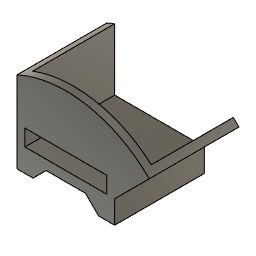
LED Mount Baffled Voron V0 V3D v7 (Autodesk Fusion 360 design; units mm, degrees)
Autodesk Fusion 360 part; units mm, degrees
note: some values were not read from the file. Set by a fixed rule: which sketch regions a step uses.
sketch "Sketch1" plane through (0, 0, 0) normal (0, 1, 0) x (1, 0, 0)
  line L0 (0, 0) -> (3, 0)
  line L1 (3, 0) -> (3, -16.2727) construction
  line L2 (9.25, -4) -> (-3.25, -4)
  line L3 (-3.25, -4) -> (-3.25, -1.5)
  line L4 (-3.25, -1.5) -> (9.25, -1.5)
  line L5 (9.25, -1.5) -> (9.25, -4)
  line L6 (9.25, -4) -> (-3.25, -1.5) construction
  line L7 (-3.25, -4) -> (9.25, -1.5) construction
  line L8 (0, 0) -> (-2, 2)
  line L9 (-2, 2) -> (-4.45, 2)
  line L10 (-4.45, 2) -> (-4.45, -1.5)
  line L11 (6, 0) -> (3, 0)
  line L12 (6, 0) -> (8, 2)
  line L13 (8, 2) -> (10.45, 2)
  line L14 (10.45, 2) -> (10.45, -1.5)
  line L15 (10.45, -1.5) -> (15.7279, -6.7779)
  arc A0 (-4.45, -10.4359) -> (15.7279, -6.7779) centre (3, 5.95) ccw
  line L16 (-4.45, -1.5) -> (-4.45, -10.4359)
  point P0 (3, -2.75)
  dimension "d3" = 2.5
  dimension "d5" = 12.5
  dimension "d9" = 135
  dimension "d10" = 2
  dimension "d11" = 1.5
  dimension "d12" = 1.2
  dimension "d14" = 3
  dimension "d20" = 18
  dimension "d21" = 45
  constraint coincident L0.start L8.start
  constraint horizontal L0
  constraint horizontal L2
  constraint perpendicular L2 L3
  constraint parallel L2 L4
  constraint parallel L3 L5
  constraint coincident L6 P0
  constraint coincident L7 P0
  constraint coincident L1 P0
  constraint horizontal L9
  constraint perpendicular L9 L10
  constraint vertical L1
  constraint coincident L4 L10.end
  constraint symmetric L0.start L1 L11.start
  constraint symmetric L0.end L1 L11.end
  constraint symmetric L1 L8.end L12.end
  constraint symmetric L1 L9.end L13.end
  constraint symmetric L1 L10.end L14.end
  constraint coincident L1 A0.centre
  constraint parallel L10 L16
  constraint coincident L15 A0.centre
  measures "d3" distance of L2.start L4.end
  measures "d5" distance of L3.end L4.end
  measures "d9" angle of L0 L8
  measures "d10" distance of L0 L9
  measures "d11" distance of L0 L4
  measures "d12" distance of L3 L10
  measures "d14" distance of L0.start L0.end
  measures "d20" radius of A0
  measures "d21" angle of L1 L15
extrude "Extrude1" add sketch "Sketch1" along normal blind 1.2
sketch "Sketch2" plane through (0, 1.2, 0) normal (0, 1, 0) x (-1, 0, 0)
  line L0 (3.25, 1.5) -> (-9.25, 1.5)
  line L1 (-9.25, 1.5) -> (-9.25, 4)
  line L2 (-9.25, 4) -> (3.25, 4)
  line L3 (3.25, 4) -> (3.25, 1.5)
  line L4 (0, 0) -> (2, -2)
  line L5 (2, -2) -> (4.45, -2)
  line L6 (4.45, -2) -> (4.45, 10.4359)
  line L7 (-15.7279, 6.7779) -> (-10.45, 1.5)
  line L8 (-10.45, 1.5) -> (-10.45, -2)
  line L9 (-10.45, -2) -> (-8, -2)
  line L10 (-8, -2) -> (-6, 0)
  line L11 (-6, 0) -> (0, 0)
  line L12 (-13.5347, 6.2818) -> (-14.8511, 7.5981)
  line L13 (-9.25, 1.9971) -> (-9.25, 1.5)
  line L14 (-9.25, 1.5) -> (3.25, 1.5)
  line L15 (3.25, 1.5) -> (3.25, 1.9971)
  line L16 (-8.4971, -0.8) -> (-6.4971, 1.2) construction
  line L17 (-6.4971, 1.2) -> (0.4971, 1.2) construction
  line L18 (0.4971, 1.2) -> (2.4971, -0.8) construction
  line L19 (2.4971, -0.8) -> (3.25, -0.8)
  line L20 (3.25, -0.8) -> (3.25, 1.9971) construction
  line L21 (-13.5347, 6.2818) -> (-9.25, 1.9971)
  line L22 (-9.25, 1.9971) -> (-9.25, -0.8) construction
  line L23 (-9.25, -0.8) -> (-8.4971, -0.8)
  arc A0 (4.45, 10.4359) -> (-15.7279, 6.7779) centre (-3, -5.95) ccw
  arc A1 (3.9533, 9.3435) -> (-14.8794, 5.9294) centre (-3, -5.95) ccw
  line L24 (3.25, 1.5) -> (3.25, 10.9301)
  dimension "d22" = 1.2
  dimension "d24" = -1.2
  constraint parallel L12 L21
  constraint coincident L0.end L1.start
  constraint coincident L0.start L3.end
  constraint parallel L10 L16
  constraint parallel L11 L17
  constraint parallel L4 L18
  constraint parallel L5 L19
  constraint parallel L6 L20
  constraint parallel L7 L21
  constraint parallel L8 L22
  constraint parallel L9 L23
  constraint coincident L12.end A0
  constraint coincident A0 L24.end
  constraint perpendicular L14 L24
  measures "d22" distance of L7 L21
extrude "Extrude2" add sketch "Sketch2" along normal blind 12.5 contours L0 L1 L3 L4 L5 L6 L7 L8 L9 L10 L11 L12 L13 L14 L15 L21 A0 A1 L24 | L7 L12 A0 A1
